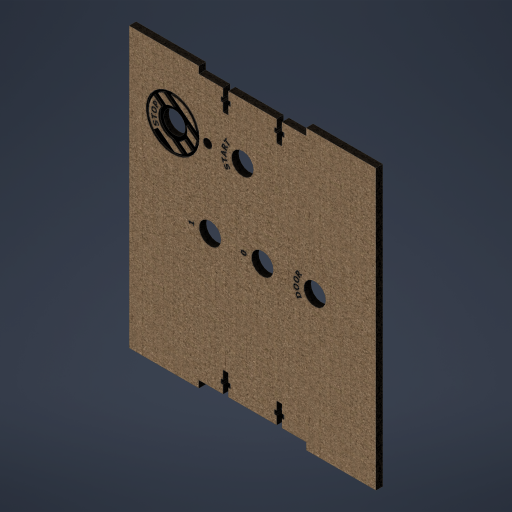
# Autodesk Inventor part: Panel
Saved by Autodesk Inventor 2024.1 (Build 281209000, 209)
## iProperties
Created: 2023-08-05
Part Number: Panel
Material: MDF Medium Density Fiberboard
Document SubType Name: Modeling
Designer: jaege
Density: 0.8 g/cm^3
Appearance: Cardboard - Corrugated
Author: jaege
Autodesk Inventor part; units mm, degrees
(part 1 of 2)
ref_plane "YZ Plane" through (0, 0, 0) normal (1, 0, 0) x (0, 1, 0)
ref_plane "XZ Plane" through (0, 0, 0) normal (0, 1, 0) x (-1, 0, 0)
ref_plane "XY Plane" through (0, 0, 0) normal (0, 0, 1) x (1, 0, 0)
sketch "Sketch1" plane through (0, 0, 0) normal (0, 0, 1) x (1, 0, 0)
  line L0 (-102.1049, 156) -> (-62.1049, 156) construction
  line L1 (-62.1049, 156) -> (-62.1049, 160) projected
  line L2 (-102.1049, 160) -> (-62.1049, 160) projected
  line L3 (-102.1049, 156) -> (-102.1049, 160) projected
  line L4 (-0.6946, 156) -> (39.3054, 156) construction
  line L5 (39.3054, 156) -> (39.3054, 160) projected
  line L6 (-0.6946, 160) -> (39.3054, 160) projected
  line L7 (-0.6946, 156) -> (-0.6946, 160) projected
  line L8 (-102.1049, 0) -> (-62.1049, 0) projected
  line L9 (-62.1049, 0) -> (-62.1049, 4) projected
  line L10 (-102.1049, 4) -> (-62.1049, 4) construction
  line L11 (-102.1049, 0) -> (-102.1049, 4) projected
  line L12 (-102.1049, 156) -> (-62.1049, 156) construction
  line L13 (39.3054, 156) -> (39.3054, 4)
  line L14 (-102.1049, 4) -> (-102.1049, 156)
  line L15 (-62.1049, 156) -> (-48.2523, 156)
  line L16 (-0.6946, 156) -> (39.3054, 156) construction
  line L17 (-0.6946, 4) -> (-62.1049, 4)
  line L18 (-62.1049, 4) -> (-102.1049, 4) construction
  line L19 (-48.2523, 156) -> (-45.2523, 156)
  line L20 (-45.2523, 156) -> (-45.2523, 144)
  line L21 (-45.2523, 144) -> (-48.2523, 144)
  line L22 (-48.2523, 144) -> (-48.2523, 156)
  line L23 (-49.4523, 148.8) -> (-44.0523, 148.8)
  line L24 (-44.0523, 148.8) -> (-44.0523, 151.2)
  line L25 (-44.0523, 151.2) -> (-49.4523, 151.2)
  line L26 (-49.4523, 151.2) -> (-49.4523, 148.8)
  line L27 (-17.5472, 156) -> (-14.5472, 156)
  line L28 (-14.5472, 156) -> (-14.5472, 144)
  line L29 (-14.5472, 144) -> (-17.5472, 144)
  line L30 (-17.5472, 144) -> (-17.5472, 156)
  line L31 (-18.7472, 148.8) -> (-13.3472, 148.8)
  line L32 (-13.3472, 148.8) -> (-13.3472, 151.2)
  line L33 (-13.3472, 151.2) -> (-18.7472, 151.2)
  line L34 (-18.7472, 151.2) -> (-18.7472, 148.8)
  line L35 (-48.2523, 16) -> (-45.2523, 16)
  line L36 (-45.2523, 16) -> (-45.2523, 4)
  line L37 (-45.2523, 4) -> (-48.2523, 4)
  line L38 (-48.2523, 4) -> (-48.2523, 16)
  line L39 (-49.4523, 8.8) -> (-44.0523, 8.8)
  line L40 (-44.0523, 8.8) -> (-44.0523, 11.2)
  line L41 (-44.0523, 11.2) -> (-49.4523, 11.2)
  line L42 (-49.4523, 11.2) -> (-49.4523, 8.8)
  line L43 (-17.5472, 16) -> (-14.5472, 16)
  line L44 (-14.5472, 16) -> (-14.5472, 4)
  line L45 (-14.5472, 4) -> (-17.5472, 4)
  line L46 (-17.5472, 4) -> (-17.5472, 16)
  line L47 (-18.7472, 8.8) -> (-13.3472, 8.8)
  line L48 (-13.3472, 8.8) -> (-13.3472, 11.2)
  line L49 (-13.3472, 11.2) -> (-18.7472, 11.2)
  line L50 (-18.7472, 11.2) -> (-18.7472, 8.8)
  line L51 (-48.2523, 0) -> (-45.2523, 0) projected
  line L52 (-17.5472, 0) -> (-14.5472, 0) projected
  line L53 (-48.2523, 156) -> (-45.2523, 156)
  line L54 (-45.2523, 156) -> (-0.6946, 156)
  line L55 (-0.6946, 0) -> (39.3054, 0) projected
  line L56 (39.3054, 0) -> (39.3054, 4) projected
  line L57 (-0.6946, 4) -> (39.3054, 4) construction
  line L58 (-0.6946, 0) -> (-0.6946, 4) projected
  point P0 (-46.7523, 151.2)
  point P1 (-46.7523, 144)
  point P2 (-46.7523, 16)
  point P3 (-46.7523, 11.2)
  point P4 (-16.0472, 156)
  point P5 (-16.0472, 151.2)
  point P6 (-16.0472, 16)
  point P7 (-16.0472, 11.2)
  point P8 (-49.4523, 150)
  point P9 (-48.2523, 150)
  point P10 (-18.7472, 150)
  point P11 (-17.5472, 150)
  point P12 (-49.4523, 10)
  point P13 (-48.2523, 10)
  point P14 (-18.7472, 10)
  point P15 (-17.5472, 10)
  point P16 (-46.7523, 0)
  point P17 (-16.0472, 0)
  point P18 (-48.2523, 4)
  point P19 (-48.2523, 8.8)
  point P20 (-48.2523, 11.2)
  point P21 (-45.2523, 11.2)
  point P22 (-45.2523, 8.8)
  point P23 (-45.2523, 4)
  point P24 (-17.5472, 4)
  point P25 (-17.5472, 8.8)
  point P26 (-17.5472, 11.2)
  point P27 (-14.5472, 11.2)
  point P28 (-14.5472, 8.8)
  point P29 (-14.5472, 4)
  point P30 (-14.5472, 151.2)
  point P31 (-14.5472, 148.8)
  point P32 (-17.5472, 148.8)
  point P33 (-17.5472, 151.2)
  point P34 (-45.2523, 151.2)
  point P35 (-45.2523, 148.8)
  point P36 (-48.2523, 148.8)
  point P37 (-48.2523, 151.2)
  dimension "d2" = 3
  dimension "d3" = 12
  dimension "d4" = 5.4
  dimension "d5" = 2.4
  dimension "d6" = 3
  dimension "d7" = 12
  dimension "d8" = 5.4
  dimension "d9" = 2.4
  dimension "d10" = 3
  dimension "d11" = 12
  dimension "d12" = 5.4
  dimension "d13" = 2.4
  dimension "d14" = 3
  dimension "d15" = 12
  dimension "d16" = 5.4
  dimension "d17" = 2.4
  constraints: 85 end point, 27 parallel, 18 midpoint, 13 horizontal, 13 perpendicular, 8 vertical alignment, 7 horizontal alignment
  measures "d2" distance of L20.end L21.end
  measures "d3" distance of L19.end L20.end
  measures "d4" distance of L25.end L24.end
  measures "d5" distance of L24.end L23.end
  measures "d6" distance of L29.start L29.end
  measures "d7" distance of L28.start L29.start
  measures "d8" distance of L34.start L33.start
  measures "d9" distance of L33.start L31.end
  measures "d10" distance of L37.start L37.end
  measures "d11" distance of L36.start L37.start
  measures "d12" distance of L42.start L41.start
  measures "d13" distance of L41.start L39.end
  measures "d14" distance of L45.start L45.end
  measures "d15" distance of L44.start L45.start
  measures "d16" distance of L50.start L49.start
  measures "d17" distance of L49.start L47.end
extrude "Extrusion1" add sketch "Sketch1" along normal blind 4 contours L15 L22 L25 L26 L23 L21 L20 L24 L54 L30 L33 L34 L31 L29 L28 L32 L7 L6 L5 L13 L56 L55 L58 L17 L44 L47 L48 L49 L43 L46 L50 L36 L39 L40 L41 L35 L38 L42 L9 L8 L11 L14 L3 L2 L1
sketch "Sketch2" plane through (0, 0, 4) normal (0, 0, 1) x (1, 0, 0)
  circle A0 centre (-77.1049, 124) radius 6.25
  circle A1 centre (-37.1049, 124) radius 6.25
  circle A2 centre (-55.6946, 80) radius 6.25
  circle A3 centre (-25.6946, 80) radius 6.25
  circle A4 centre (4.3054, 80) radius 6.25
  circle A5 centre (-57.1049, 124) radius 2.5
  line L0 (-77.1049, 124) -> (-57.1049, 124) construction
  line L1 (-57.1049, 124) -> (-37.1049, 124) construction
  line L2 (-45.2523, 144) -> (-48.2523, 144) projected
  line L3 (-55.6946, 80) -> (-25.6946, 80) construction
  line L4 (-25.6946, 80) -> (4.3054, 80) construction
  line L5 (-102.1049, 160) -> (-102.1049, 0) projected
  line L6 (39.3054, 0) -> (39.3054, 160) projected
  point P0 (-46.7523, 144)
  point P1 (-47.1049, 124)
  point P2 (39.3054, 80)
  dimension "d18" = 12.5
  dimension "d21" = 5
  dimension "d23" = 20
  dimension "d24" = 20
  dimension "d25" = 30
  dimension "d29" = 25
  dimension "d30" = 35
  constraints: 8 end point, 6 centre point, 4 collinear, 4 equal radius, 4 horizontal alignment, 3 midpoint, 2 horizontal
  measures "d18" diameter of A0
  measures "d21" diameter of A5
  measures "d23" distance of L0.start L0.end
  measures "d24" vertical distance of point (-46.752, 144) point (-47.105, 124)
  measures "d25" distance of L3.start L3.end
  measures "d29" distance from line of L5 L0.start
  measures "d30" distance of point (39.305, 80) L4.end
extrude "Extrusion2" cut sketch "Sketch2" against normal up to next
sketch "Sketch3" plane through (0, 0, 4) normal (0, 0, 1) x (1, 0, 0)
  circle A0 centre (-37.1049, 124) radius 6.25 construction
  circle A1 centre (4.3054, 80) radius 6.25 construction
  circle A2 centre (-57.1049, 124) radius 2.5 construction
  circle A3 centre (-55.6946, 80) radius 6.25 construction
  circle A4 centre (-25.6946, 80) radius 6.25 construction
  circle A5 centre (-77.1049, 124) radius 6.25 construction
  line L0 (-62.1049, 156) -> (-62.1049, 160) construction
  line L1 (-62.1049, 160) -> (-102.1049, 160) construction
  line L2 (-102.1049, 160) -> (-102.1049, 0) construction
  line L3 (-102.1049, 0) -> (-62.1049, 0) construction
  line L4 (-62.1049, 0) -> (-62.1049, 4) construction
  line L5 (-62.1049, 4) -> (-48.2523, 4) construction
  line L6 (-48.2523, 4) -> (-48.2523, 8.8) construction
  line L7 (-48.2523, 8.8) -> (-49.4523, 8.8) construction
  line L8 (-49.4523, 8.8) -> (-49.4523, 11.2) construction
  line L9 (-49.4523, 11.2) -> (-48.2523, 11.2) construction
  line L10 (-48.2523, 11.2) -> (-48.2523, 16) construction
  line L11 (-48.2523, 16) -> (-45.2523, 16) construction
  line L12 (-45.2523, 16) -> (-45.2523, 11.2) construction
  line L13 (-45.2523, 11.2) -> (-44.0523, 11.2) construction
  line L14 (-44.0523, 11.2) -> (-44.0523, 8.8) construction
  line L15 (-44.0523, 8.8) -> (-45.2523, 8.8) construction
  line L16 (-45.2523, 8.8) -> (-45.2523, 4) construction
  line L17 (-45.2523, 4) -> (-17.5472, 4) construction
  line L18 (-17.5472, 4) -> (-17.5472, 8.8) construction
  line L19 (-17.5472, 8.8) -> (-18.7472, 8.8) construction
  line L20 (-18.7472, 8.8) -> (-18.7472, 11.2) construction
  line L21 (-18.7472, 11.2) -> (-17.5472, 11.2) construction
  line L22 (-17.5472, 11.2) -> (-17.5472, 16) construction
  line L23 (-17.5472, 16) -> (-14.5472, 16) construction
  line L24 (-14.5472, 16) -> (-14.5472, 11.2) construction
  line L25 (-14.5472, 11.2) -> (-13.3472, 11.2) construction
  line L26 (-13.3472, 11.2) -> (-13.3472, 8.8) construction
  line L27 (-13.3472, 8.8) -> (-14.5472, 8.8) construction
  line L28 (-14.5472, 8.8) -> (-14.5472, 4) construction
  line L29 (-14.5472, 4) -> (-0.6946, 4) construction
  line L30 (-0.6946, 4) -> (-0.6946, 0) construction
  line L31 (-0.6946, 0) -> (39.3054, 0) construction
  line L32 (39.3054, 0) -> (39.3054, 160) construction
  line L33 (39.3054, 160) -> (-0.6946, 160) construction
  line L34 (-0.6946, 160) -> (-0.6946, 156) construction
  line L35 (-0.6946, 156) -> (-14.5472, 156) construction
  line L36 (-14.5472, 156) -> (-14.5472, 151.2) construction
  line L37 (-14.5472, 151.2) -> (-13.3472, 151.2) construction
  line L38 (-13.3472, 151.2) -> (-13.3472, 148.8) construction
  line L39 (-13.3472, 148.8) -> (-14.5472, 148.8) construction
  line L40 (-14.5472, 148.8) -> (-14.5472, 144) construction
  line L41 (-14.5472, 144) -> (-17.5472, 144) construction
  line L42 (-17.5472, 144) -> (-17.5472, 148.8) construction
  line L43 (-17.5472, 148.8) -> (-18.7472, 148.8) construction
  line L44 (-18.7472, 148.8) -> (-18.7472, 151.2) construction
  line L45 (-18.7472, 151.2) -> (-17.5472, 151.2) construction
  line L46 (-17.5472, 151.2) -> (-17.5472, 156) construction
  line L47 (-17.5472, 156) -> (-45.2523, 156) construction
  line L48 (-45.2523, 156) -> (-45.2523, 151.2) construction
  line L49 (-45.2523, 151.2) -> (-44.0523, 151.2) construction
  line L50 (-44.0523, 151.2) -> (-44.0523, 148.8) construction
  line L51 (-44.0523, 148.8) -> (-45.2523, 148.8) construction
  line L52 (-45.2523, 148.8) -> (-45.2523, 144) construction
  line L53 (-45.2523, 144) -> (-48.2523, 144) construction
  line L54 (-48.2523, 144) -> (-48.2523, 148.8) construction
  line L55 (-48.2523, 148.8) -> (-49.4523, 148.8) construction
  line L56 (-49.4523, 148.8) -> (-49.4523, 151.2) construction
  line L57 (-49.4523, 151.2) -> (-48.2523, 151.2) construction
  line L58 (-48.2523, 151.2) -> (-48.2523, 156) construction
  line L59 (-48.2523, 156) -> (-62.1049, 156) construction
  circle A6 centre (-77.1049, 124) radius 13.75
  circle A7 centre (-77.1049, 124) radius 8.25
  spline S0 degree 2 poles (-85.3183, 119.8642) (-85.1628, 119.5496) (-85.0505, 119.0151) (-85.0384, 118.7675) knots 0 0 0 1 2 2 2
  line L60 (-85.0384, 118.7675) -> (-85.6899, 118.4456)
  line L61 (-85.6899, 118.4456) -> (-85.7206, 118.5077)
  spline S1 degree 2 poles (-85.7206, 118.5077) (-85.6473, 118.8002) (-85.703, 119.3875) (-85.818, 119.6201) knots 0 0 0 1 2 2 2
  spline S2 degree 2 poles (-85.818, 119.6201) (-85.8475, 119.68) (-85.9694, 119.8596) (-86.0244, 119.9041) knots 0 0 0 1 2 2 2
  spline S3 degree 2 poles (-86.0244, 119.9041) (-86.0905, 119.9597) (-86.2527, 120.0036) (-86.3436, 119.9587) knots 0 0 0 1 2 2 2
  spline S4 degree 2 poles (-86.3436, 119.9587) (-86.4478, 119.9073) (-86.4964, 119.682) (-86.4704, 119.557) knots 0 0 0 1 2 2 2
  spline S5 degree 2 poles (-86.4704, 119.557) (-86.4392, 119.3988) (-86.3469, 119.0501) (-86.3267, 118.8864) knots 0 0 0 1 2 2 2
  spline S6 degree 2 poles (-86.3267, 118.8864) (-86.2809, 118.5148) (-86.5241, 118.0528) (-86.8078, 117.9127) knots 0 0 0 1 2 2 2
  spline S7 degree 2 poles (-86.8078, 117.9127) (-87.1912, 117.7233) (-87.9883, 118.1373) (-88.2292, 118.6248) knots 0 0 0 1 2 2 2
  spline S8 degree 2 poles (-88.2292, 118.6248) (-88.3496, 118.8686) (-88.4885, 119.4009) (-88.4984, 119.6331) knots 0 0 0 1 2 2 2
  line L62 (-88.4984, 119.6331) -> (-87.8735, 119.9418)
  line L63 (-87.8735, 119.9418) -> (-87.8439, 119.882)
  spline S9 degree 2 poles (-87.8439, 119.882) (-87.8992, 119.6645) (-87.8619, 119.137) (-87.7481, 118.9066) knots 0 0 0 1 2 2 2
  spline S10 degree 2 poles (-87.7481, 118.9066) (-87.7032, 118.8157) (-87.6065, 118.687) (-87.5317, 118.6248) knots 0 0 0 1 2 2 2
  spline S11 degree 2 poles (-87.5317, 118.6248) (-87.4711, 118.5747) (-87.3099, 118.5386) (-87.239, 118.5736) knots 0 0 0 1 2 2 2
  spline S12 degree 2 poles (-87.239, 118.5736) (-87.1326, 118.6261) (-87.0841, 118.8348) (-87.1404, 119.0716) knots 0 0 0 1 2 2 2
  spline S13 degree 2 poles (-87.1404, 119.0716) (-87.1773, 119.2244) (-87.2433, 119.5088) (-87.2646, 119.6802) knots 0 0 0 1 2 2 2
  spline S14 degree 2 poles (-87.2646, 119.6802) (-87.3006, 120.0153) (-87.0917, 120.4631) (-86.8081, 120.6032) knots 0 0 0 1 2 2 2
  spline S15 degree 2 poles (-86.8081, 120.6032) (-86.4003, 120.8046) (-85.5876, 120.4094) (-85.3183, 119.8642) knots 0 0 0 1 2 2 2
  line L64 (-86.1407, 121.9842) -> (-88.5708, 121.5467)
  line L65 (-88.5708, 121.5467) -> (-88.411, 120.6588)
  line L66 (-88.411, 120.6588) -> (-88.9826, 120.5559)
  line L67 (-88.9826, 120.5559) -> (-89.438, 123.0858)
  line L68 (-89.438, 123.0858) -> (-88.8664, 123.1887)
  line L69 (-88.8664, 123.1887) -> (-88.7065, 122.3008)
  line L70 (-88.7065, 122.3008) -> (-86.2764, 122.7383)
  line L71 (-86.2764, 122.7383) -> (-86.1407, 121.9842)
  spline S16 degree 2 poles (-87.5894, 126.8908) (-86.8544, 126.7926) (-86.1189, 125.8964) (-86.2099, 125.2153) knots 0 0 0 1 2 2 2
  spline S17 degree 2 poles (-86.2099, 125.2153) (-86.3012, 124.5318) (-87.2554, 123.8664) (-87.9806, 123.9632) knots 0 0 0 1 2 2 2
  spline S18 degree 2 poles (-87.9806, 123.9632) (-88.7082, 124.0605) (-89.4517, 124.9528) (-89.3604, 125.6363) knots 0 0 0 1 2 2 2
  spline S19 degree 2 poles (-89.3604, 125.6363) (-89.2694, 126.3174) (-88.3219, 126.9887) (-87.5894, 126.8908) knots 0 0 0 1 2 2 2
  spline S20 degree 2 poles (-87.6941, 126.1069) (-87.9661, 126.1432) (-88.3605, 126.0837) (-88.4933, 126.0042) knots 0 0 0 1 2 2 2
  spline S21 degree 2 poles (-88.4933, 126.0042) (-88.631, 125.9254) (-88.7716, 125.6948) (-88.7893, 125.5625) knots 0 0 0 1 2 2 2
  spline S22 degree 2 poles (-88.7893, 125.5625) (-88.8079, 125.4228) (-88.7379, 125.1816) (-88.6246, 125.0592) knots 0 0 0 1 2 2 2
  spline S23 degree 2 poles (-88.6246, 125.0592) (-88.5194, 124.9504) (-88.1453, 124.7832) (-87.8758, 124.7472) knots 0 0 0 1 2 2 2
  spline S24 degree 2 poles (-87.8758, 124.7472) (-87.5965, 124.7099) (-87.2143, 124.771) (-87.0766, 124.8499) knots 0 0 0 1 2 2 2
  spline S25 degree 2 poles (-87.0766, 124.8499) (-86.9389, 124.9287) (-86.798, 125.1618) (-86.7804, 125.2941) knots 0 0 0 1 2 2 2
  spline S26 degree 2 poles (-86.7804, 125.2941) (-86.7624, 125.4288) (-86.8441, 125.6941) (-86.9545, 125.8011) knots 0 0 0 1 2 2 2
  spline S27 degree 2 poles (-86.9545, 125.8011) (-87.0737, 125.9167) (-87.41, 126.0689) (-87.6941, 126.1069) knots 0 0 0 1 2 2 2
  spline S28 degree 2 poles (-86.7343, 130.1226) (-86.5432, 130.0295) (-86.2562, 129.7383) (-86.1959, 129.5687) knots 0 0 0 1 2 2 2
  spline S29 degree 2 poles (-86.1959, 129.5687) (-86.1561, 129.4641) (-86.1185, 129.2367) (-86.125, 129.1162) knots 0 0 0 1 2 2 2
  spline S30 degree 2 poles (-86.125, 129.1162) (-86.1326, 128.9934) (-86.1996, 128.7319) (-86.2711, 128.5852) knots 0 0 0 1 2 2 2
  line L72 (-86.2711, 128.5852) -> (-86.4465, 128.2253)
  line L73 (-86.4465, 128.2253) -> (-85.549, 127.7878)
  line L74 (-85.549, 127.7878) -> (-85.8847, 127.099)
  line L75 (-85.8847, 127.099) -> (-88.6263, 128.4355)
  line L76 (-88.6263, 128.4355) -> (-88.1075, 129.4997)
  spline S31 degree 2 poles (-88.1075, 129.4997) (-87.9927, 129.7352) (-87.7382, 130.0373) (-87.5767, 130.1318) knots 0 0 0 1 2 2 2
  spline S32 degree 2 poles (-87.5767, 130.1318) (-87.3964, 130.2364) (-86.972, 130.2385) (-86.7343, 130.1226) knots 0 0 0 1 2 2 2
  spline S33 degree 2 poles (-87.0609, 129.4074) (-87.1786, 129.4648) (-87.3994, 129.435) (-87.4674, 129.3746) knots 0 0 0 1 2 2 2
  spline S34 degree 2 poles (-87.4674, 129.3746) (-87.5572, 129.2974) (-87.6572, 129.1262) (-87.7319, 128.9729) knots 0 0 0 1 2 2 2
  line L77 (-87.7319, 128.9729) -> (-87.7796, 128.8751)
  line L78 (-87.7796, 128.8751) -> (-86.9575, 128.4744)
  line L79 (-86.9575, 128.4744) -> (-86.9337, 128.5233)
  spline S35 degree 2 poles (-86.9337, 128.5233) (-86.8871, 128.6188) (-86.8071, 128.7943) (-86.7868, 128.8641) knots 0 0 0 1 2 2 2
  spline S36 degree 2 poles (-86.7868, 128.8641) (-86.7686, 128.924) (-86.7624, 129.0722) (-86.7795, 129.1218) knots 0 0 0 1 2 2 2
  spline S37 degree 2 poles (-86.7795, 129.1218) (-86.8114, 129.2253) (-86.9365, 129.3468) (-87.0609, 129.4074) knots 0 0 0 1 2 2 2
  point P0 (0, 0)
  dimension "d31" = 7.5
  dimension "d32" = 2
  constraints: 2 centre point, 1 other
  measures "d31" radial gap between concentric circles of A5 A6
  measures "d32" radial gap between concentric circles of A5 A7
emboss "Emboss1" sketch "Sketch3" operation cut depth 1 direction (0, 0, -1) contours S0 L60 L61 S1 S2 S3 S4 S5 S6 S7 S8 L62 L63 S9 S10 S11 S12 S13 S14 S15 | L64 L65 L66 L67 L68 L69 L70 L71 | S16 S17 S18 S19 | S28 S29 S30 L72 L73 L74 L75 L76 S31 S32
sketch "Sketch4" plane through (0, 0, 4) normal (0, 0, 1) x (1, 0, 0)
  line L0 (-88.7065, 122.3008) -> (-86.2764, 122.7383) construction
  line L1 (-86.2764, 122.7383) -> (-86.1407, 121.9842) construction
  line L2 (-86.1407, 121.9842) -> (-88.5708, 121.5467) construction
  line L3 (-88.5708, 121.5467) -> (-88.411, 120.6588) construction
  line L4 (-88.411, 120.6588) -> (-88.9826, 120.5559) construction
  line L5 (-88.9826, 120.5559) -> (-89.438, 123.0858) construction
  line L6 (-89.438, 123.0858) -> (-88.8664, 123.1887) construction
  line L7 (-88.8664, 123.1887) -> (-88.7065, 122.3008) construction
  line L8 (-87.8735, 119.9418) -> (-87.8439, 119.882) construction
  line L9 (-85.0384, 118.7675) -> (-85.6899, 118.4456) construction
  line L10 (-85.6899, 118.4456) -> (-85.7206, 118.5077) construction
  line L11 (-88.4984, 119.6331) -> (-87.8735, 119.9418) construction
  line L12 (-85.8847, 127.099) -> (-88.6263, 128.4355) construction
  line L13 (-88.6263, 128.4355) -> (-88.1075, 129.4997) construction
  line L14 (-86.2711, 128.5852) -> (-86.4465, 128.2253) construction
  line L15 (-86.4465, 128.2253) -> (-85.549, 127.7878) construction
  line L16 (-85.549, 127.7878) -> (-85.8847, 127.099) construction
  circle A0 centre (-37.1049, 124) radius 6.25 construction
  circle A1 centre (4.3054, 80) radius 6.25 construction
  circle A2 centre (-57.1049, 124) radius 2.5 construction
  circle A3 centre (-55.6946, 80) radius 6.25 construction
  circle A4 centre (-25.6946, 80) radius 6.25 construction
  circle A5 centre (-77.1049, 124) radius 6.25 construction
  line L17 (-62.1049, 156) -> (-62.1049, 160) construction
  line L18 (-62.1049, 160) -> (-102.1049, 160) construction
  line L19 (-102.1049, 160) -> (-102.1049, 0) construction
  line L20 (-102.1049, 0) -> (-62.1049, 0) construction
  line L21 (-62.1049, 0) -> (-62.1049, 4) construction
  line L22 (-62.1049, 4) -> (-48.2523, 4) construction
  line L23 (-48.2523, 4) -> (-48.2523, 8.8) construction
  line L24 (-48.2523, 8.8) -> (-49.4523, 8.8) construction
  line L25 (-49.4523, 8.8) -> (-49.4523, 11.2) construction
  line L26 (-49.4523, 11.2) -> (-48.2523, 11.2) construction
  line L27 (-48.2523, 11.2) -> (-48.2523, 16) construction
  line L28 (-48.2523, 16) -> (-45.2523, 16) construction
  line L29 (-45.2523, 16) -> (-45.2523, 11.2) construction
  line L30 (-45.2523, 11.2) -> (-44.0523, 11.2) construction
  line L31 (-44.0523, 11.2) -> (-44.0523, 8.8) construction
  line L32 (-44.0523, 8.8) -> (-45.2523, 8.8) construction
  line L33 (-45.2523, 8.8) -> (-45.2523, 4) construction
  line L34 (-45.2523, 4) -> (-17.5472, 4) construction
  line L35 (-17.5472, 4) -> (-17.5472, 8.8) construction
  line L36 (-17.5472, 8.8) -> (-18.7472, 8.8) construction
  line L37 (-18.7472, 8.8) -> (-18.7472, 11.2) construction
  line L38 (-18.7472, 11.2) -> (-17.5472, 11.2) construction
  line L39 (-17.5472, 11.2) -> (-17.5472, 16) construction
  line L40 (-17.5472, 16) -> (-14.5472, 16) construction
  line L41 (-14.5472, 16) -> (-14.5472, 11.2) construction
  line L42 (-14.5472, 11.2) -> (-13.3472, 11.2) construction
  line L43 (-13.3472, 11.2) -> (-13.3472, 8.8) construction
  line L44 (-13.3472, 8.8) -> (-14.5472, 8.8) construction
  line L45 (-14.5472, 8.8) -> (-14.5472, 4) construction
  line L46 (-14.5472, 4) -> (-0.6946, 4) construction
  line L47 (-0.6946, 4) -> (-0.6946, 0) construction
  line L48 (-0.6946, 0) -> (39.3054, 0) construction
  line L49 (39.3054, 0) -> (39.3054, 160) construction
  line L50 (39.3054, 160) -> (-0.6946, 160) construction
  line L51 (-0.6946, 160) -> (-0.6946, 156) construction
  line L52 (-0.6946, 156) -> (-14.5472, 156) construction
  line L53 (-14.5472, 156) -> (-14.5472, 151.2) construction
  line L54 (-14.5472, 151.2) -> (-13.3472, 151.2) construction
  line L55 (-13.3472, 151.2) -> (-13.3472, 148.8) construction
  line L56 (-13.3472, 148.8) -> (-14.5472, 148.8) construction
  line L57 (-14.5472, 148.8) -> (-14.5472, 144) construction
  line L58 (-14.5472, 144) -> (-17.5472, 144) construction
  line L59 (-17.5472, 144) -> (-17.5472, 148.8) construction
  line L60 (-17.5472, 148.8) -> (-18.7472, 148.8) construction
  line L61 (-18.7472, 148.8) -> (-18.7472, 151.2) construction
  line L62 (-18.7472, 151.2) -> (-17.5472, 151.2) construction
  line L63 (-17.5472, 151.2) -> (-17.5472, 156) construction
  line L64 (-17.5472, 156) -> (-45.2523, 156) construction
  line L65 (-45.2523, 156) -> (-45.2523, 151.2) construction
  line L66 (-45.2523, 151.2) -> (-44.0523, 151.2) construction
  line L67 (-44.0523, 151.2) -> (-44.0523, 148.8) construction
  line L68 (-44.0523, 148.8) -> (-45.2523, 148.8) construction
  line L69 (-45.2523, 148.8) -> (-45.2523, 144) construction
  line L70 (-45.2523, 144) -> (-48.2523, 144) construction
  line L71 (-48.2523, 144) -> (-48.2523, 148.8) construction
  line L72 (-48.2523, 148.8) -> (-49.4523, 148.8) construction
  line L73 (-49.4523, 148.8) -> (-49.4523, 151.2) construction
  line L74 (-49.4523, 151.2) -> (-48.2523, 151.2) construction
  line L75 (-48.2523, 151.2) -> (-48.2523, 156) construction
  line L76 (-48.2523, 156) -> (-62.1049, 156) construction
  circle A6 centre (-77.1049, 124) radius 8.25
  circle A7 centre (-77.1049, 124) radius 13.75
  line L77 (-88.0135, 115.6295) -> (-83.6501, 118.9777)
  line L78 (-77.1049, 124) -> (-83.6501, 118.9777) construction
  line L79 (-77.1049, 124) -> (-83.6501, 129.0223) construction
  line L80 (-83.6501, 129.0223) -> (-88.0135, 132.3705)
  line L81 (-77.1049, 124) -> (-90.8549, 124) construction
  line L82 (-74.5667, 104.7209) -> (-96.384, 121.4619)
  line L83 (-96.384, 121.4619) -> (-94.2913, 124.189)
  line L84 (-94.2913, 124.189) -> (-72.4741, 107.4481)
  line L85 (-72.4741, 107.4481) -> (-74.5667, 104.7209)
  line L86 (-92.1987, 126.9162) -> (-70.3815, 110.1752)
  line L87 (-70.3815, 110.1752) -> (-68.2889, 112.9024)
  line L88 (-68.2889, 112.9024) -> (-90.1061, 129.6433)
  line L89 (-90.1061, 129.6433) -> (-92.1987, 126.9162)
  line L90 (-66.1963, 115.6295) -> (-88.0135, 132.3705)
  line L91 (-88.0135, 132.3705) -> (-85.9209, 135.0976)
  line L92 (-85.9209, 135.0976) -> (-64.1037, 118.3567)
  line L93 (-64.1037, 118.3567) -> (-66.1963, 115.6295)
  line L94 (-83.8283, 137.8248) -> (-62.011, 121.0838)
  line L95 (-62.011, 121.0838) -> (-59.9184, 123.811)
  line L96 (-59.9184, 123.811) -> (-81.7356, 140.5519)
  line L97 (-81.7356, 140.5519) -> (-83.8283, 137.8248)
  line L98 (-94.2913, 124.189) -> (-92.1987, 126.9162)
  line L99 (-90.1061, 129.6433) -> (-88.0135, 132.3705)
  line L100 (-85.9209, 135.0976) -> (-83.8283, 137.8248)
  line L101 (-66.1963, 115.6295) -> (-74.5667, 104.7209)
  line L102 (-88.0135, 132.3705) -> (-96.384, 121.4619)
  circle A8 centre (-77.1049, 124) radius 15.25
  circle A9 centre (-55.6946, 80) radius 8.25 construction
  circle A10 centre (-25.6946, 80) radius 8.25 construction
  circle A11 centre (4.3054, 80) radius 8.25 construction
  circle A12 centre (-37.1049, 124) radius 8.25 construction
  line L103 (-81.7356, 140.5519) -> (-59.9184, 123.811)
  line L104 (-59.9184, 123.811) -> (-57.8258, 126.5381)
  line L105 (-57.8258, 126.5381) -> (-79.643, 143.2791)
  line L106 (-79.643, 143.2791) -> (-81.7356, 140.5519)
  line L107 (-64.9446, 81.0789) -> (-64.9446, 79.0645)
  line L108 (-64.9446, 79.0645) -> (-65.476, 79.0645)
  line L109 (-65.476, 79.0645) -> (-65.476, 79.7071)
  line L110 (-65.476, 79.7071) -> (-67.09, 79.7071)
  line L111 (-67.09, 79.7071) -> (-67.09, 79.0645)
  line L112 (-67.09, 79.0645) -> (-67.5868, 79.0645)
  spline S0 degree 2 poles (-67.5868, 79.0645) (-67.5868, 79.2054) (-67.6238, 79.4847) (-67.6634, 79.5687) knots 0 0 0 1 2 2 2
  spline S1 degree 2 poles (-67.6634, 79.5687) (-67.7128, 79.6651) (-67.8784, 79.7738) (-68.002, 79.7837) knots 0 0 0 1 2 2 2
  line L113 (-68.002, 79.7837) -> (-68.002, 80.4511)
  line L114 (-68.002, 80.4511) -> (-65.476, 80.4511)
  line L115 (-65.476, 80.4511) -> (-65.476, 81.0789)
  line L116 (-65.476, 81.0789) -> (-64.9446, 81.0789)
  spline S2 degree 2 poles (-36.4696, 81.1753) (-36.0741, 81.1753) (-35.4809, 81.0492) (-35.2807, 80.9083) knots 0 0 0 1 2 2 2
  spline S3 degree 2 poles (-35.2807, 80.9083) (-35.083, 80.7699) (-34.8803, 80.3225) (-34.8803, 80.0012) knots 0 0 0 1 2 2 2
  spline S4 degree 2 poles (-34.8803, 80.0012) (-34.8803, 79.6775) (-35.083, 79.2326) (-35.2857, 79.0917) knots 0 0 0 1 2 2 2
  spline S5 degree 2 poles (-35.2857, 79.0917) (-35.4859, 78.9508) (-36.0741, 78.8247) (-36.4696, 78.8247) knots 0 0 0 1 2 2 2
  spline S6 degree 2 poles (-36.4696, 78.8247) (-36.8749, 78.8247) (-37.4484, 78.9508) (-37.656, 79.0941) knots 0 0 0 1 2 2 2
  spline S7 degree 2 poles (-37.656, 79.0941) (-37.8587, 79.2375) (-38.0564, 79.6898) (-38.0564, 80.0012) knots 0 0 0 1 2 2 2
  spline S8 degree 2 poles (-38.0564, 80.0012) (-38.0564, 80.33) (-37.8488, 80.7699) (-37.6436, 80.9108) knots 0 0 0 1 2 2 2
  spline S9 degree 2 poles (-37.6436, 80.9108) (-37.4434, 81.0492) (-36.8527, 81.1753) (-36.4696, 81.1753) knots 0 0 0 1 2 2 2
  spline S10 degree 2 poles (-36.4696, 80.4066) (-37.0356, 80.4066) (-37.4929, 80.2212) (-37.4929, 80.0012) knots 0 0 0 1 2 2 2
  spline S11 degree 2 poles (-37.4929, 80.0012) (-37.4929, 79.7813) (-37.0356, 79.5934) (-36.4671, 79.5934) knots 0 0 0 1 2 2 2
  spline S12 degree 2 poles (-36.4671, 79.5934) (-35.9085, 79.5934) (-35.4439, 79.7813) (-35.4439, 80.0012) knots 0 0 0 1 2 2 2
  spline S13 degree 2 poles (-35.4439, 80.0012) (-35.4439, 80.2187) (-35.9085, 80.4066) (-36.4696, 80.4066) knots 0 0 0 1 2 2 2
  spline S14 degree 2 poles (-5.8084, 76.0175) (-5.435, 76.2258) (-4.666, 76.2275) (-4.37, 76.0671) knots 0 0 0 1 2 2 2
  spline S15 degree 2 poles (-4.37, 76.0671) (-4.1206, 75.9346) (-3.7707, 75.4901) (-3.6178, 75.216) knots 0 0 0 1 2 2 2
  line L117 (-3.6178, 75.216) -> (-3.153, 74.3828)
  line L118 (-3.153, 74.3828) -> (-5.8165, 72.8969)
  line L119 (-5.8165, 72.8969) -> (-6.2765, 73.7214)
  spline S16 degree 2 poles (-6.2765, 73.7214) (-6.433, 74.002) (-6.6352, 74.5317) (-6.6174, 74.8246) knots 0 0 0 1 2 2 2
  spline S17 degree 2 poles (-6.6174, 74.8246) (-6.5948, 75.1797) (-6.1947, 75.802) (-5.8084, 76.0175) knots 0 0 0 1 2 2 2
  spline S18 degree 2 poles (-5.4298, 75.3287) (-5.6931, 75.1818) (-5.9675, 74.791) (-5.9697, 74.5463) knots 0 0 0 1 2 2 2
  spline S19 degree 2 poles (-5.9697, 74.5463) (-5.9672, 74.3694) (-5.8162, 74.0631) (-5.7006, 73.8559) knots 0 0 0 1 2 2 2
  line L120 (-5.7006, 73.8559) -> (-5.6933, 73.843)
  line L121 (-5.6933, 73.843) -> (-4.0249, 74.7738)
  line L122 (-4.0249, 74.7738) -> (-4.0321, 74.7867)
  spline S20 degree 2 poles (-4.0321, 74.7867) (-4.1573, 75.0112) (-4.3446, 75.3115) (-4.5114, 75.4024) knots 0 0 0 1 2 2 2
  spline S21 degree 2 poles (-4.5114, 75.4024) (-4.7065, 75.5086) (-5.1664, 75.4756) (-5.4298, 75.3287) knots 0 0 0 1 2 2 2
  spline S22 degree 2 poles (-6.5655, 79.6762) (-5.8342, 79.7987) (-4.8674, 79.1587) (-4.7539, 78.481) knots 0 0 0 1 2 2 2
  spline S23 degree 2 poles (-4.7539, 78.481) (-4.6399, 77.8009) (-5.3559, 76.8841) (-6.0775, 76.7632) knots 0 0 0 1 2 2 2
  spline S24 degree 2 poles (-6.0775, 76.7632) (-6.8015, 76.6419) (-7.7748, 77.2758) (-7.8887, 77.9559) knots 0 0 0 1 2 2 2
  spline S25 degree 2 poles (-7.8887, 77.9559) (-8.0022, 78.6335) (-7.2944, 79.5541) (-6.5655, 79.6762) knots 0 0 0 1 2 2 2
  spline S26 degree 2 poles (-6.4348, 78.8961) (-6.7054, 78.8508) (-7.0649, 78.6778) (-7.1684, 78.5627) knots 0 0 0 1 2 2 2
  spline S27 degree 2 poles (-7.1684, 78.5627) (-7.2768, 78.4468) (-7.3432, 78.1851) (-7.3211, 78.0535) knots 0 0 0 1 2 2 2
  spline S28 degree 2 poles (-7.3211, 78.0535) (-7.2979, 77.9145) (-7.1599, 77.7046) (-7.0156, 77.621) knots 0 0 0 1 2 2 2
  spline S29 degree 2 poles (-7.0156, 77.621) (-6.8831, 77.5479) (-6.4763, 77.4983) (-6.2082, 77.5432) knots 0 0 0 1 2 2 2
  spline S30 degree 2 poles (-6.2082, 77.5432) (-5.9303, 77.5898) (-5.583, 77.7607) (-5.4746, 77.8766) knots 0 0 0 1 2 2 2
  spline S31 degree 2 poles (-5.4746, 77.8766) (-5.3662, 77.9925) (-5.3002, 78.2567) (-5.3223, 78.3883) knots 0 0 0 1 2 2 2
  spline S32 degree 2 poles (-5.3223, 78.3883) (-5.3447, 78.5224) (-5.5009, 78.7518) (-5.6379, 78.8216) knots 0 0 0 1 2 2 2
  spline S33 degree 2 poles (-5.6379, 78.8216) (-5.7859, 78.8971) (-6.1521, 78.9435) (-6.4348, 78.8961) knots 0 0 0 1 2 2 2
  spline S34 degree 2 poles (-6.0319, 83.3795) (-5.3024, 83.2469) (-4.6097, 82.3172) (-4.7325, 81.6411) knots 0 0 0 1 2 2 2
  spline S35 degree 2 poles (-4.7325, 81.6411) (-4.8558, 80.9627) (-5.8402, 80.3427) (-6.56, 80.4735) knots 0 0 0 1 2 2 2
  spline S36 degree 2 poles (-6.56, 80.4735) (-7.2823, 80.6048) (-7.9831, 81.531) (-7.8598, 82.2094) knots 0 0 0 1 2 2 2
  spline S37 degree 2 poles (-7.8598, 82.2094) (-7.737, 82.8855) (-6.759, 83.5116) (-6.0319, 83.3795) knots 0 0 0 1 2 2 2
  spline S38 degree 2 poles (-6.1733, 82.6013) (-6.4433, 82.6504) (-6.8401, 82.6095) (-6.9765, 82.5363) knots 0 0 0 1 2 2 2
  spline S39 degree 2 poles (-6.9765, 82.5363) (-7.1177, 82.464) (-7.2689, 82.2402) (-7.2928, 82.1089) knots 0 0 0 1 2 2 2
  spline S40 degree 2 poles (-7.2928, 82.1089) (-7.318, 81.9703) (-7.2594, 81.726) (-7.1519, 81.5985) knots 0 0 0 1 2 2 2
  spline S41 degree 2 poles (-7.1519, 81.5985) (-7.052, 81.4849) (-6.6861, 81.3003) (-6.4186, 81.2517) knots 0 0 0 1 2 2 2
  spline S42 degree 2 poles (-6.4186, 81.2517) (-6.1414, 81.2013) (-5.7567, 81.2444) (-5.6155, 81.3168) knots 0 0 0 1 2 2 2
  spline S43 degree 2 poles (-5.6155, 81.3168) (-5.4742, 81.3891) (-5.3226, 81.6152) (-5.2987, 81.7465) knots 0 0 0 1 2 2 2
  spline S44 degree 2 poles (-5.2987, 81.7465) (-5.2744, 81.8803) (-5.3436, 82.1491) (-5.4489, 82.2612) knots 0 0 0 1 2 2 2
  spline S45 degree 2 poles (-5.4489, 82.2612) (-5.5625, 82.3823) (-5.8912, 82.5501) (-6.1733, 82.6013) knots 0 0 0 1 2 2 2
  line L123 (-2.9465, 85.964) -> (-3.4061, 85.1534)
  line L124 (-3.4061, 85.1534) -> (-4.7982, 84.9682)
  line L125 (-4.7982, 84.9682) -> (-4.9347, 84.7273)
  line L126 (-4.9347, 84.7273) -> (-3.9607, 84.1751)
  line L127 (-3.9607, 84.1751) -> (-4.3362, 83.5129)
  line L128 (-4.3362, 83.5129) -> (-6.9894, 85.0172)
  line L129 (-6.9894, 85.0172) -> (-6.3848, 86.0836)
  spline S46 degree 2 poles (-6.3848, 86.0836) (-6.2592, 86.3051) (-6.018, 86.6002) (-5.8528, 86.6912) knots 0 0 0 1 2 2 2
  spline S47 degree 2 poles (-5.8528, 86.6912) (-5.682, 86.7819) (-5.3053, 86.7899) (-5.0903, 86.668) knots 0 0 0 1 2 2 2
  spline S48 degree 2 poles (-5.0903, 86.668) (-4.7871, 86.4961) (-4.5626, 86.0052) (-4.5812, 85.7117) knots 0 0 0 1 2 2 2
  line L130 (-4.5812, 85.7117) -> (-2.9465, 85.964)
  spline S49 degree 2 poles (-5.394, 85.9368) (-5.4951, 85.994) (-5.683, 85.9983) (-5.7717, 85.9321) knots 0 0 0 1 2 2 2
  spline S50 degree 2 poles (-5.7717, 85.9321) (-5.8329, 85.8844) (-5.9345, 85.7403) (-5.9991, 85.6263) knots 0 0 0 1 2 2 2
  line L131 (-5.9991, 85.6263) -> (-6.1259, 85.4027)
  line L132 (-6.1259, 85.4027) -> (-5.412, 84.998)
  line L133 (-5.412, 84.998) -> (-5.3035, 85.1893)
  spline S51 degree 2 poles (-5.3035, 85.1893) (-5.2255, 85.3269) (-5.149, 85.5421) (-5.165, 85.6392) knots 0 0 0 1 2 2 2
  spline S52 degree 2 poles (-5.165, 85.6392) (-5.18, 85.733) (-5.2822, 85.8734) (-5.394, 85.9368) knots 0 0 0 1 2 2 2
  spline S53 degree 2 poles (-44.6829, 118.7906) (-44.4863, 118.4999) (-44.3027, 117.9856) (-44.2572, 117.7418) knots 0 0 0 1 2 2 2
  line L134 (-44.2572, 117.7418) -> (-44.8591, 117.3348)
  line L135 (-44.8591, 117.3348) -> (-44.8979, 117.3921)
  spline S54 degree 2 poles (-44.8979, 117.3921) (-44.8649, 117.6919) (-44.9996, 118.2662) (-45.145, 118.4812) knots 0 0 0 1 2 2 2
  spline S55 degree 2 poles (-45.145, 118.4812) (-45.1824, 118.5364) (-45.3274, 118.698) (-45.388, 118.7346) knots 0 0 0 1 2 2 2
  spline S56 degree 2 poles (-45.388, 118.7346) (-45.4609, 118.7807) (-45.6277, 118.8022) (-45.7116, 118.7455) knots 0 0 0 1 2 2 2
  spline S57 degree 2 poles (-45.7116, 118.7455) (-45.8078, 118.6804) (-45.8255, 118.4506) (-45.7829, 118.3303) knots 0 0 0 1 2 2 2
  spline S58 degree 2 poles (-45.7829, 118.3303) (-45.7305, 118.1777) (-45.5919, 117.8448) (-45.5497, 117.6853) knots 0 0 0 1 2 2 2
  spline S59 degree 2 poles (-45.5497, 117.6853) (-45.4541, 117.3233) (-45.6325, 116.8327) (-45.8946, 116.6555) knots 0 0 0 1 2 2 2
  spline S60 degree 2 poles (-45.8946, 116.6555) (-46.2488, 116.416) (-47.0947, 116.7182) (-47.3993, 117.1686) knots 0 0 0 1 2 2 2
  spline S61 degree 2 poles (-47.3993, 117.1686) (-47.5516, 117.3939) (-47.7613, 117.9025) (-47.8025, 118.1312) knots 0 0 0 1 2 2 2
  line L136 (-47.8025, 118.1312) -> (-47.2251, 118.5216)
  line L137 (-47.2251, 118.5216) -> (-47.1878, 118.4663)
  spline S62 degree 2 poles (-47.1878, 118.4663) (-47.213, 118.2434) (-47.1047, 117.7258) (-46.9608, 117.5129) knots 0 0 0 1 2 2 2
  spline S63 degree 2 poles (-46.9608, 117.5129) (-46.904, 117.429) (-46.7908, 117.3145) (-46.7082, 117.263) knots 0 0 0 1 2 2 2
  spline S64 degree 2 poles (-46.7082, 117.263) (-46.6414, 117.2216) (-46.4768, 117.2076) (-46.4113, 117.2519) knots 0 0 0 1 2 2 2
  spline S65 degree 2 poles (-46.4113, 117.2519) (-46.313, 117.3184) (-46.2932, 117.5317) (-46.381, 117.7587) knots 0 0 0 1 2 2 2
  spline S66 degree 2 poles (-46.381, 117.7587) (-46.4382, 117.905) (-46.5422, 118.1779) (-46.5864, 118.3449) knots 0 0 0 1 2 2 2
  spline S67 degree 2 poles (-46.5864, 118.3449) (-46.6674, 118.672) (-46.5211, 119.1439) (-46.259, 119.3211) knots 0 0 0 1 2 2 2
  spline S68 degree 2 poles (-46.259, 119.3211) (-45.8823, 119.5759) (-45.0235, 119.2943) (-44.6829, 118.7906) knots 0 0 0 1 2 2 2
  line L138 (-45.7847, 120.7797) -> (-48.1332, 120.0174)
  line L139 (-48.1332, 120.0174) -> (-47.8547, 119.1593)
  line L140 (-47.8547, 119.1593) -> (-48.4072, 118.98)
  line L141 (-48.4072, 118.98) -> (-49.2008, 121.4249)
  line L142 (-49.2008, 121.4249) -> (-48.6483, 121.6043)
  line L143 (-48.6483, 121.6043) -> (-48.3698, 120.7462)
  line L144 (-48.3698, 120.7462) -> (-46.0213, 121.5085)
  line L145 (-46.0213, 121.5085) -> (-45.7847, 120.7797)
  line L146 (-46.323, 122.3501) -> (-49.3935, 123.318)
  line L147 (-49.3935, 123.318) -> (-49.4106, 124.1533)
  line L148 (-49.4106, 124.1533) -> (-46.3824, 125.2462)
  line L149 (-46.3824, 125.2462) -> (-46.3662, 124.4579)
  line L150 (-46.3662, 124.4579) -> (-46.985, 124.2549)
  line L151 (-46.985, 124.2549) -> (-46.9654, 123.2961)
  line L152 (-46.9654, 123.2961) -> (-46.3387, 123.1161)
  line L153 (-46.3387, 123.1161) -> (-46.323, 122.3501)
  line L154 (-47.5351, 124.0755) -> (-48.537, 123.7435)
  line L155 (-48.537, 123.7435) -> (-47.5223, 123.4503)
  line L156 (-47.5223, 123.4503) -> (-47.5351, 124.0755)
  line L157 (-45.4742, 128.2561) -> (-45.7477, 127.3653)
  line L158 (-45.7477, 127.3653) -> (-47.0669, 126.8836)
  line L159 (-47.0669, 126.8836) -> (-47.1482, 126.619)
  line L160 (-47.1482, 126.619) -> (-46.0779, 126.2903)
  line L161 (-46.0779, 126.2903) -> (-46.3014, 125.5626)
  line L162 (-46.3014, 125.5626) -> (-49.217, 126.458)
  line L163 (-49.217, 126.458) -> (-48.8571, 127.6299)
  spline S69 degree 2 poles (-48.8571, 127.6299) (-48.7823, 127.8733) (-48.6106, 128.2135) (-48.469, 128.3381) knots 0 0 0 1 2 2 2
  spline S70 degree 2 poles (-48.469, 128.3381) (-48.3218, 128.4635) (-47.9557, 128.5528) (-47.7194, 128.4802) knots 0 0 0 1 2 2 2
  spline S71 degree 2 poles (-47.7194, 128.4802) (-47.3863, 128.3779) (-47.061, 127.947) (-47.0157, 127.6565) knots 0 0 0 1 2 2 2
  line L164 (-47.0157, 127.6565) -> (-45.4742, 128.2561)
  spline S72 degree 2 poles (-47.858, 127.7006) (-47.9691, 127.7347) (-48.1535, 127.6982) (-48.2258, 127.6144) knots 0 0 0 1 2 2 2
  spline S73 degree 2 poles (-48.2258, 127.6144) (-48.2752, 127.5546) (-48.3432, 127.3919) (-48.3817, 127.2667) knots 0 0 0 1 2 2 2
  line L165 (-48.3817, 127.2667) -> (-48.4572, 127.021)
  line L166 (-48.4572, 127.021) -> (-47.6727, 126.7801)
  line L167 (-47.6727, 126.7801) -> (-47.6082, 126.9904)
  spline S74 degree 2 poles (-47.6082, 126.9904) (-47.5617, 127.1416) (-47.5335, 127.3682) (-47.5701, 127.4596) knots 0 0 0 1 2 2 2
  spline S75 degree 2 poles (-47.5701, 127.4596) (-47.605, 127.5479) (-47.7352, 127.6628) (-47.858, 127.7006) knots 0 0 0 1 2 2 2
  line L168 (-44.9597, 128.9002) -> (-46.9987, 130.2927)
  line L169 (-46.9987, 130.2927) -> (-47.5075, 129.5477)
  line L170 (-47.5075, 129.5477) -> (-47.9871, 129.8752)
  line L171 (-47.9871, 129.8752) -> (-46.5375, 131.998)
  line L172 (-46.5375, 131.998) -> (-46.0578, 131.6704)
  line L173 (-46.0578, 131.6704) -> (-46.5666, 130.9254)
  line L174 (-46.5666, 130.9254) -> (-44.5276, 129.5329)
  line L175 (-44.5276, 129.5329) -> (-44.9597, 128.9002)
  point P0 (0, 0)
  point P1 (-89.7597, 129.3775)
  point P2 (-85.1474, 125.8384)
  point P3 (-69.0623, 122.1616)
  point P4 (-85.5745, 134.8318)
  point P5 (-83.6501, 129.0223)
  point P6 (-63.4725, 122.2053)
  point P7 (-82.3668, 136.7033)
  point P8 (-64.4501, 118.6225)
  point P9 (-80.9622, 131.2927)
  point P10 (-70.5597, 118.9777)
  point P11 (-68.6353, 113.1682)
  point P12 (-73.2476, 116.7073)
  point P13 (-77.6721, 115.7695)
  point P14 (-71.843, 111.2967)
  point P15 (-76.1674, 110.282)
  point P16 (-85.575, 117.5007)
  point P17 (-68.2889, 112.9024)
  point P18 (-92.0286, 127.1379)
  point P19 (-90.7079, 117.1064)
  point P20 (-83.9984, 137.603)
  point P21 (-83.7191, 137.741)
  point P22 (-70.2113, 110.397)
  point P23 (-70.4907, 110.259)
  point P24 (-78.0424, 137.718)
  point P25 (-63.6117, 126.6449)
  point P26 (-69.3017, 126.6781)
  point P27 (-76.5376, 132.2305)
  point P28 (-92.0896, 126.8324)
  dimension "d38" = 2
  dimension "d39" = 7.5
  dimension "d40" = 75
  dimension "d44" = 1.5
  dimension "d45" = 2
  dimension "d46" = 2
  dimension "d47" = 2
  dimension "d48" = 2
  constraints: 60 end point, 17 collinear, 11 parallel, 8 perpendicular, 7 centre point, 7 point on circle, 6 point on line, 4 tangent, 1 horizontal, 30 other
  measures "d38" radial gap between concentric circles of A5 A6
  measures "d39" radial gap between concentric circles of A5 A7
  measures "d40" angle of L79 L78
  measures "d44" radial gap between concentric circles of A7 A8
  measures "d45" radial gap between concentric circles of A3 A9
  measures "d46" radial gap between concentric circles of A4 A10
  measures "d47" radial gap between concentric circles of A1 A11
  measures "d48" radial gap between concentric circles of A0 A12
extrude "Extrusion3" cut sketch "Sketch4" against normal blind 1 contours A6 L92 L94 | L94 A6 | A6 L94 A7 L96 | L92 A7 L90 A6 | A6 L90 L92 | L94 A8 L87 L101 L93 L92 A7 | A7 L96 A8 L94 | A6 L88 L90 | A6 L80 A7 L92 | L92 L93 A7 | L94 A8 L96 A7 | A7 L92 L100 A8 L94 | L88 A7 L86 A6 | A6 L86 L88 | L101 L88 A7 | A7 L91 L92 | L96 A8 L105 A7 | A7 L105 A8 L96 | A8 L86 A7 L88 L87 | A6 L86 | L99 L89 A8 L100 L91 | A7 L88 L99 | L105 A8 | A8 L84 A7 L86 | A7 L86 A8 L89 L88 | A8 L82 A7 L84 | L84 A7 L77 | A7 L84 A8 L86 | A8 L82 | A7 L82 A8 L84 | L107 L108 L109 L110 L111 L112 S0 S1 L113 L114 L115 L116 | S2 S3 S4 S5 S6 S7 S8 S9 | S14 S15 L117 L118 L119 S16 S17 | S22 S23 S24 S25 | S34 S35 S36 S37 | L123 L124 L125 L126 L127 L128 L129 S46 S47 S48 L130 | S53 L134 L135 S54 S55 S56 S57 S58 S59 S60 S61 L136 L137 S62 S63 S64 S65 S66 S67 S68 | L138 L139 L140 L141 L142 L143 L144 L145 | L146 L147 L148 L149 L150 L151 L152 L153 | L157 L158 L159 L160 L161 L162 L163 S69 S70 S71 L164 | L168 L169 L170 L171 L172 L173 L174 L175 picked at (-73.2488, 114.7086) picked at (-80.4032, 112.7457)